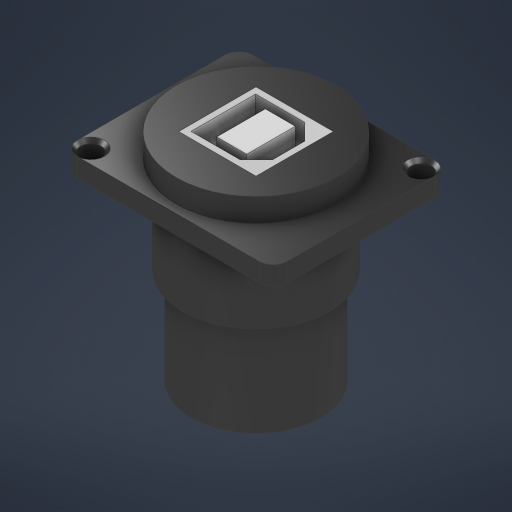
# Autodesk Inventor part: USB Type B Socket
Saved by Autodesk Inventor 2024 (Build 280153000, 153)
## iProperties
Created: 2025-11-26
Part Number: USB Type B Socket
Material: Generic
Document SubType Name: Modeling
Designer: Vincent Larson
Density: 1 g/cm^3
Appearance: Default
Author: Vincent Larson
Autodesk Inventor part; units mm, degrees
ref_plane "YZ Plane" through (0, 0, 0) normal (1, 0, 0) x (0, 1, 0)
ref_plane "XZ Plane" through (0, 0, 0) normal (0, 1, 0) x (-1, 0, 0)
ref_plane "XY Plane" through (0, 0, 0) normal (0, 0, 1) x (1, 0, 0)
sketch "Sketch1" plane through (0, 0, 0) normal (0, 1, 0) x (-1, 0, 0)
  line L0 (-15.494, 12.954) -> (15.494, 12.954)
  line L1 (15.494, 12.954) -> (15.494, -12.954)
  line L2 (15.494, -12.954) -> (-15.494, -12.954)
  line L3 (-15.494, -12.954) -> (-15.494, 12.954)
  line L4 (-15.494, 12.954) -> (15.494, -12.954) construction
  line L5 (15.494, 12.954) -> (-15.494, -12.954) construction
  line L6 (15.494, 12.954) -> (0, 0)
  line L7 (15.494, 12.954) -> (13.462, 12.954)
  line L8 (13.462, 12.954) -> (13.462, 10.922)
  line L9 (13.462, 10.922) -> (15.494, 10.922)
  circle A0 centre (13.462, 10.922) radius 2.032
  line L10 (-15.494, -12.954) -> (-13.462, -12.954)
  line L11 (-13.462, -12.954) -> (-13.462, -10.922)
  line L12 (-13.462, -10.922) -> (-15.494, -10.922)
  line L13 (-15.494, -10.922) -> (-15.494, -12.954)
  line L14 (-15.494, 12.954) -> (-13.462, 12.954)
  line L15 (-13.462, 12.954) -> (-13.462, 10.922)
  line L16 (-13.462, 10.922) -> (-15.494, 10.922)
  line L17 (-15.494, 10.922) -> (-15.494, 12.954)
  line L18 (15.494, -12.954) -> (13.462, -12.954)
  line L19 (13.462, -12.954) -> (13.462, -10.922)
  line L20 (13.462, -10.922) -> (15.494, -10.922)
  line L21 (15.494, -10.922) -> (15.494, -12.954)
  circle A1 centre (13.462, -10.922) radius 2.032
  circle A2 centre (-13.462, 10.922) radius 2.032
  circle A3 centre (-13.462, -10.922) radius 2.032
  circle A4 centre (-13.462, 10.922) radius 1.5367
  circle A5 centre (13.462, 10.922) radius 1.5367
  circle A6 centre (13.462, -10.922) radius 1.5367
  circle A7 centre (-13.462, -10.922) radius 1.5367
  dimension "d0" = 30.988
  dimension "d1" = 25.908
  dimension "d2" = 2.032
  dimension "d3" = 2.032
  dimension "d4" = 2.032
  dimension "d5" = 2.032
  dimension "d6" = 3.0734
  constraints: 44 end point, 8 coincident, 8 parallel, 6 perpendicular, 5 centre point, 4 horizontal, 4 point on line, 2 midpoint, 1 collinear, 1 tangent, 9 other
  measures "d0" distance of L1.end L2.end
  measures "d1" distance of L0.end L1.end
  measures "d2" distance of L0.end L7.end
  measures "d3" distance of L7.end L8.end
  measures "d4" distance of L12.end L11.end
  measures "d5" distance of L11.end L10.end
  measures "d6" diameter of A4
extrude "Extrusion1" add sketch "Sketch1" along normal blind 2.794 contours A2 L16 A4 L15 | L0 A0 L1 A1 L2 A3 L3 A2 | L15 A4 L16 A2 | A0 L6 A5 L8 | L8 A5 L6 A0 | A3 L11 A7 L12 | L12 A7 L11 A3 | A0 L9 A5 L6 | L6 A5 L9 A0 | A1 L20 A6 L19 | L19 A6 L20 A1
sketch "Sketch2" plane through (0, 2.794, 0) normal (0, 1, 0) x (1, 0, 0)
  circle A0 centre (-13.462, 10.922) radius 1.5367 projected
  circle A1 centre (-13.462, 10.922) radius 1.5367
  circle A2 centre (13.462, -10.922) radius 1.5367 projected
  circle A3 centre (13.462, -10.922) radius 1.5367
  point P0 (0, 0)
  constraints: 2 centre point, 2 coincident
extrude "Extrusion2" add sketch "Sketch2" against normal blind 2.794
sketch "Sketch3" plane through (0, 2.794, 0) normal (0, 1, 0) x (1, 0, 0)
  circle A0 centre (0, 0) radius 11.7856
  dimension "d11" = 23.5712
  constraints: 1 centre point, 1 coincident
  measures "d11" diameter of A0
extrude "Extrusion3" add sketch "Sketch3" along normal blind 3.429
sketch "Sketch4" plane through (0, 0, 0) normal (0, -1, 0) x (1, 0, 0)
  circle A0 centre (0, 0) radius 10.8712
  dimension "d14" = 21.7424
  constraints: 1 centre point, 1 coincident
  measures "d14" diameter of A0
extrude "Extrusion4" add sketch "Sketch4" along normal blind 11.3792
sketch "Sketch5" plane through (0, -11.3792, 0) normal (0, -1, 0) x (1, 0, 0)
  circle A0 centre (0, 0) radius 9.5631
  dimension "d17" = 19.1262
  constraints: 1 centre point, 1 coincident
  measures "d17" diameter of A0
extrude "Extrusion5" add sketch "Sketch5" along normal blind 14.2494
sketch "Sketch6" plane through (0, 6.223, 0) normal (0, 1, 0) x (1, 0, 0)
  line L0 (5.715, -5.715) -> (-5.715, -5.715)
  line L1 (-5.715, -5.715) -> (-5.715, 5.715)
  line L2 (-5.715, 5.715) -> (5.715, 5.715)
  line L3 (5.715, 5.715) -> (5.715, -5.715)
  line L4 (5.715, -5.715) -> (-5.715, 5.715) construction
  line L5 (-5.715, -5.715) -> (5.715, 5.715) construction
  point P0 (0, 0)
  dimension "d20" = 11.43
  dimension "d21" = 11.43
  constraints: 12 end point, 2 midpoint, 2 parallel, 1 horizontal, 1 perpendicular
  measures "d20" distance of L1.end L2.end
  measures "d21" distance of L0.end L1.end
extrude "Extrusion6" cut sketch "Sketch6" against normal blind 0.0254
sketch "Sketch7" plane through (0, 6.1976, 0) normal (0, 1, 0) x (1, 0, 0)
  line L0 (4.8156, -4.768) -> (-4.8156, -4.768)
  line L1 (-4.8156, -4.768) -> (-4.8156, 4.768)
  line L2 (-4.8156, 4.768) -> (4.8156, 4.768)
  line L3 (4.8156, 4.768) -> (4.8156, -4.768)
  line L4 (4.8156, -4.768) -> (-4.8156, 4.768) construction
  line L5 (-4.8156, -4.768) -> (4.8156, 4.768) construction
  line L6 (4.8156, -4.768) -> (4.8156, 0)
  line L7 (4.8156, -2.384) -> (2.4316, -4.768)
  line L8 (4.8156, -2.384) -> (8.1872, -2.384) construction
  line L9 (4.8156, 0) -> (4.8156, 4.768)
  line L10 (4.8156, 2.384) -> (2.4316, 4.768)
  line L11 (4.8156, 2.384) -> (8.1872, 2.384) construction
  point P0 (0, 0)
  dimension "d24" = 135
  dimension "d25" = 135
  constraints: 24 end point, 5 midpoint, 3 horizontal, 2 equal length, 2 parallel, 2 point on line, 1 collinear, 1 perpendicular
  measures "d24" angle of L7 L8
  measures "d25" angle of L11 L10
extrude "Extrusion7" cut sketch "Sketch7" against normal blind 8.89 contours L0 L1 L2 L10 L3 L7
sketch "Sketch8" plane through (0, -2.6924, 0) normal (0, 1, 0) x (1, 0, 0)
  line L0 (-2.2203, -3.589) -> (2.2203, -3.589)
  line L1 (2.2203, -3.589) -> (2.2203, 3.589)
  line L2 (2.2203, 3.589) -> (-2.2203, 3.589)
  line L3 (-2.2203, 3.589) -> (-2.2203, -3.589)
  line L4 (-2.2203, -3.589) -> (2.2203, 3.589) construction
  line L5 (2.2203, -3.589) -> (-2.2203, 3.589) construction
  point P0 (0, 0)
  constraints: 12 end point, 2 midpoint, 2 parallel, 1 horizontal, 1 perpendicular
extrude "Extrusion8" add sketch "Sketch8" along normal blind 8.89
chamfer "Chamfer1" distance 0.508 angle 45 2 edges at (-11.9253, 2.794, 10.922) (14.9987, 2.794, -10.922)
body "Solid1"
